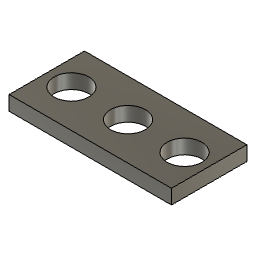
PE Filter Riser v2 (Autodesk Fusion 360 design; units mm, degrees)
Autodesk Fusion 360 part; units mm, degrees
sketch "Sketch1" plane through (0, 0, 0) normal (0, 0, 1) x (1, 0, 0) in component "Component"
  line L0 (-13, 0) -> (-13, 6.5)
  line L1 (-13, 0) -> (-13, -6.5)
  line L2 (-13, -6.5) -> (13, -6.5)
  line L3 (13, -6.5) -> (13, 6.5)
  line L4 (13, 6.5) -> (-13, 6.5)
  circle A0 centre (0, 0) radius 3
  line L5 (0, 0) -> (9.75, 0)
  line L6 (0, 0) -> (-9.75, 0)
  circle A1 centre (-9.75, 0) radius 3
  circle A2 centre (9.75, 0) radius 3
  line L7 (13, -6.5) -> (14, -6.5)
  line L8 (14, -6.5) -> (14, 6.5)
  line L9 (14, 6.5) -> (13, 6.5)
  line L10 (-13, 6.5) -> (-14, 6.5)
  line L11 (-14, 6.5) -> (-14, -6.5)
  line L12 (-14, -6.5) -> (-13, -6.5)
  dimension "d2" = 13
  dimension "d3" = 6.5
  dimension "d4" = 6.5
  dimension "d5" = 13
  dimension "d6" = 9.75
  dimension "d7" = 9.75
  dimension "d8" = 6
  dimension "d9" = 6
  dimension "d10" = 13
  dimension "d11" = 13
  constraint perpendicular L0 L2
  constraint perpendicular L2 L3
  constraint coincident A0.centre L5.start
  constraint horizontal L5
  constraint parallel L5 L6
  constraint coincident L6.end A1.centre
  constraint coincident L5.end A2.centre
  constraint perpendicular L3 L7
  constraint perpendicular L7 L8
  constraint perpendicular L3 L9
  constraint perpendicular L0 L10
  constraint perpendicular L4 L11
  constraint perpendicular L1 L12
  measures "d2" distance of A0.centre L0.start
  measures "d3" distance of L0.start L0.end
  measures "d4" distance of L0.start L1.end
  measures "d5" distance of L2.end L3.end
  measures "d6" distance of A0.centre L5.end
  measures "d7" distance of A0.centre L6.end
  measures "d8" diameter of A1
  measures "d9" diameter of A2
  measures "d10" distance of L7.end L8.end
  measures "d11" distance of L10.end L11.end
extrude "Extrude1" add sketch "Sketch1" along normal blind 2.5 in component "Component"
component "Component" placed x (1, 0, 0) y (0, 1, 0) z (0, 0, 1) at (0, 0, 0)
named bodies: "PE Filter Riser"
